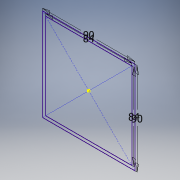
# Autodesk Inventor part: Front Motor Connector
Saved by Autodesk Inventor 2019 (Build 230136000, 136)
## iProperties
Created: 2019-10-26
Part Number: Front Motor Connector
Material: Generic
Document SubType Name: Modeling
Designer: Mark
Density: 1 g/cm^3
Appearance: Default
Author: Mark
Autodesk Inventor part; units mm, degrees
ref_plane "YZ Plane" through (0, 0, 0) normal (1, 0, 0) x (0, 1, 0)
ref_plane "XZ Plane" through (0, 0, 0) normal (0, 1, 0) x (-1, 0, 0)
ref_plane "XY Plane" through (0, 0, 0) normal (0, 0, 1) x (1, 0, 0)
sketch "Sketch1" plane through (0, 0, 0) normal (0, 0, 1) x (1, 0, 0)
  line L0 (-27.5, -45) -> (27.5, -45)
  line L1 (27.5, -45) -> (27.5, 45)
  line L2 (27.5, 45) -> (-27.5, 45)
  line L3 (-27.5, 45) -> (-27.5, -45)
  line L4 (-27.5, -45) -> (27.5, 45) construction
  line L5 (27.5, -45) -> (-27.5, 45) construction
  line L6 (-24.5, -42) -> (24.5, -42)
  line L7 (24.5, -42) -> (24.5, 42)
  line L8 (24.5, 42) -> (-24.5, 42)
  line L9 (-24.5, 42) -> (-24.5, -42)
  line L10 (-24.5, -42) -> (24.5, 42) construction
  line L11 (24.5, -42) -> (-24.5, 42) construction
  point P0 (0, 0)
  dimension "d0" = 55
  dimension "d1" = 90
  dimension "d2" = 49
  dimension "d3" = 84
  constraints: 24 end point, 4 midpoint, 4 parallel, 2 horizontal, 2 perpendicular
  measures "d0" distance of L2.end L1.end
  measures "d1" distance of L1.end L0.end
  measures "d2" distance of L8.end L7.end
  measures "d3" distance of L7.end L6.end
extrude "Extrusion1" add sketch "Sketch1" along normal blind 50
sketch "Sketch2" plane through (-27.5, -45, 0) normal (0, -1, 0) x (1, 0, 0)
  circle A0 centre (15, 40) radius 2.75
  circle A1 centre (40, 40) radius 2.75
  circle A2 centre (15, 10) radius 2.75
  circle A3 centre (40, 10) radius 2.75
  line L0 (55, 0) -> (55, 50) projected
  line L1 (0, 50) -> (55, 50) projected
  line L2 (0, 0) -> (55, 0) projected
  line L3 (0, 0) -> (0, 50) projected
  point P0 (27.5, 0)
  dimension "d6" = 5.5
  dimension "d7" = 5.5
  dimension "d8" = 5.5
  dimension "d9" = 5.5
  dimension "d10" = 15
  dimension "d11" = 10
  dimension "d12" = 15
  dimension "d13" = 10
  dimension "d14" = 10
  dimension "d15" = 15
  dimension "d16" = 15
  dimension "d17" = 10
  constraints: 4 centre point
  measures "d6" diameter of A0
  measures "d7" diameter of A1
  measures "d8" diameter of A2
  measures "d9" diameter of A3
  measures "d10" distance from line of L0 A1.centre
  measures "d11" distance from line of L1 A1.centre
  measures "d12" distance from line of L0 A3.centre
  measures "d13" distance from line of L2 A3.centre
  measures "d14" distance from line of L2 A2.centre
  measures "d15" distance from line of L3 A2.centre
  measures "d16" distance from line of L3 A0.centre
  measures "d17" distance from line of L1 A0.centre
extrude "Extrusion2" cut sketch "Sketch2" against normal blind 97.625 contours A0 | A1 | A2 | A3
body "Solid1"
